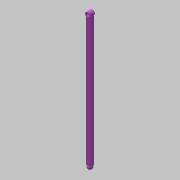
# Autodesk Inventor part: LinkRod
Saved by Autodesk Inventor 2015 (Build 190159000, 159)
## iProperties
Created: 2016-06-12
Part Number: LinkRod
Material: 一般
Document SubType Name: Modeling
Designer: kumagai
Density: 1 g/cm^3
Appearance: 既定
Author: kumagai
Autodesk Inventor part; units mm, degrees
ref_plane "YZ Plane" through (0, 0, 0) normal (1, 0, 0) x (0, 1, 0)
ref_plane "XZ Plane" through (0, 0, 0) normal (0, 1, 0) x (-1, 0, 0)
ref_plane "XY Plane" through (0, 0, 0) normal (0, 0, 1) x (1, 0, 0)
sketch "スケッチ1" plane through (0, 0, 0) normal (0, 1, 0) x (-1, 0, 0)
  line L0 (0, -331.5666) -> (0, 61.0944) projected
  line L1 (-9.0498, 0) -> (7.3416, 0) projected
  circle A0 centre (0, 0) radius 5
  circle A1 centre (0, 0) radius 3
  arc A2 (4, -267) -> (0, -275) centre (0, -270) ccw
  line L2 (4, -267) -> (4, -3)
  line L3 (-4, -267) -> (-4, -3)
  line L4 (0, -275) -> (0, -265)
  line L5 (4, -267) -> (-4, -267)
  dimension "d0" = 10
  dimension "d1" = 6
  dimension "d2" = 10
  dimension "d3" = 270
  dimension "d4" = 8
  constraints: 8 end point, 6 point on circle, 3 centre point, 3 point on line, 2 coincident, 2 parallel, 1 perpendicular, 1 other
  measures "d0" diameter of A2
  measures "d1" diameter of A1
  measures "d2" diameter of A0
  measures "d3" distance of point (0, 0) A2.centre
  measures "d4" distance between parallel lines of L3 L2
extrude "押し出し1" add sketch "スケッチ1" along normal mid plane 10 contours A0 L1 A1 L0 | L0 A1 L1 A0 | A0 L0 A1 L1 | L1 A1 L0 A0
revolve "回転1" add sketch "スケッチ1" angle 360 about axis through (0, 0, 0) along (0, 0, 1) picked at (-0.4059, -272.2831) picked at (-2.4012, -266.7204) contours A2 L5 L0 | L5 A2 L0
extrude "押し出し2" add sketch "スケッチ1" along normal mid plane 8 contours L5 A2 L0 | L0 A2 L5 | L3 A0 L0 A2 | L0 A0 L2 A2 picked at (-2.4012, -266.7204) picked at (2.4012, -266.7204)
